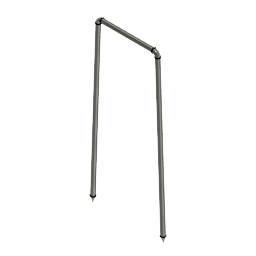
FA6 - 12 Gauge 4” Staple Stake (Autodesk Fusion 360 design; units mm, degrees)
Autodesk Fusion 360 part; units mm, degrees
sketch "Sketch1" plane through (0, 0, 0) normal (0, 1, 0) x (1, 0, 0)
  line L0 (0, 0) -> (0, -101.6) construction
  line L1 (0, -101.6) -> (16.1278, -101.6)
  line L2 (18.6263, -99.1872) -> (22.09, 0)
  line L3 (18.542, -101.6) -> (48.3661, -101.6) construction
  line L4 (0, 0) -> (22.09, 0) construction
  arc A0 (16.1278, -101.6) -> (18.6263, -99.1872) centre (16.1278, -99.1) ccw
  line L5 (0, -101.6) -> (-16.1278, -101.6)
  arc A1 (-18.6263, -99.1872) -> (-16.1278, -101.6) centre (-16.1278, -99.1) ccw
  line L6 (-18.6263, -99.1872) -> (-22.09, 0)
  line L7 (0, -101.6) -> (-18.75, -101.6) construction
  line L8 (-18.75, -101.6) -> (-18.75, -100.3) construction
  dimension "d1" = 101.6
  dimension "d2" = 18.542
  dimension "d3" = 88
  dimension "d4" = 2.5
  dimension "d13" = 18.75
  dimension "d14" = 1.3
  constraint coincident L0.start L4.start
  constraint vertical L0
  constraint perpendicular L0 L1
  constraint horizontal L3
  constraint perpendicular L0 L4
  constraint coincident L3.start L1
  constraint coincident L3.start L2
  constraint tangent L1 A0
  constraint tangent L2 A0
  constraint symmetric L1.start L0 L5.start
  constraint symmetric L0 L2.end L6.end
  constraint symmetric L0 L1.end L5.end
  constraint symmetric L0 L2.start A1.start
  constraint symmetric L0 A0 A1
  constraint perpendicular L0 L7
  constraint perpendicular L7 L8
  measures "d1" distance of L0.start L0.end
  measures "d2" distance of L0.end L3.start
  measures "d3" angle of L2 L3
  measures "d4" radius of A0
  measures "d13" distance of L0.end L7.end
  measures "d14" distance of L7.end L8.end
sketch "Sketch3" plane through (0, 0, 0) normal (1, 0, 0) x (0, 1, 0)
  line L0 (0, 0) -> (0, 101.6) construction
  circle A0 centre (0, 101.6) radius 1.3
  dimension "d5" = 101.6
  dimension "d6" = 2.6
  constraint coincident L0.start origin
  constraint vertical L0
  constraint coincident L0.end A0.centre
  measures "d5" distance of L0.start L0.end
  measures "d6" diameter of A0
sweep "Sweep1" add profiles "Sketch3" path "Sketch1" along L6 A1 L5 L1 A0 L2 section 1
ref_plane "WorkPlane1" through (0, 0, 100.3) normal (0, 0, 1) x (1, 0, 0)
sketch "Sketch4" plane through (0, 0, 100.3) normal (0, 0, 1) x (1, 0, 0)
  line L0 (0, 0) -> (-18.75, 0) construction
  circle A0 centre (-18.75, 0) radius 5 construction
  dimension "d16" = 18.75
  dimension "d17" = 10
  constraint coincident L0.start origin
  constraint horizontal L0
  constraint coincident L0.end A0.centre
  measures "d16" distance of L0.start L0.end
  measures "d17" diameter of A0
chamfer "Chamfer1" distance 1.3 distance2 4 2 edges at (-22.5598, -1.212, 0.0164) (21.6201, -1.212, -0.0164) measured on face at (-22.2737, 0.4465, 0.0064) measured on face at (22.1502, -0.4097, 0.0021)
equation "d2 = ( 37.084 / 2 ) * 1 mm"
equation "d13 = ( 37.5 / 2 ) * 1 mm"
